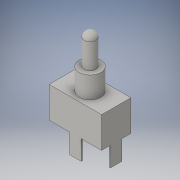
# Autodesk Inventor part: switch toggle
Saved by Autodesk Inventor 2016 (Build 200138000, 138)
## iProperties
Created: 2015-10-15
Part Number: switch toggle
Material: Generic
Document SubType Name: Modeling
Designer: jeremyhale
Density: 1 g/cm^3
Appearance: Default
Author: jeremyhale
Autodesk Inventor part; units mm, degrees
ref_plane "YZ Plane" through (0, 0, 0) normal (1, 0, 0) x (0, 1, 0)
ref_plane "XZ Plane" through (0, 0, 0) normal (0, 1, 0) x (-1, 0, 0)
ref_plane "XY Plane" through (0, 0, 0) normal (0, 0, 1) x (1, 0, 0)
sketch "Sketch1" plane through (0, 0, 0) normal (0, 1, 0) x (-1, 0, 0)
  line L0 (-14.4018, 8.0518) -> (14.4018, 8.0518)
  line L1 (14.4018, 8.0518) -> (14.4018, -8.0518)
  line L2 (14.4018, -8.0518) -> (-14.4018, -8.0518)
  line L3 (-14.4018, -8.0518) -> (-14.4018, 8.0518)
  line L4 (-14.4018, 8.0518) -> (14.4018, -8.0518) construction
  line L5 (14.4018, 8.0518) -> (-14.4018, -8.0518) construction
  point P0 (0, 0)
  dimension "d0" = 28.8036
  dimension "d1" = 16.1036
  constraints: 12 end point, 2 midpoint, 2 parallel, 1 horizontal, 1 perpendicular
  measures "d0" distance of L1.end L2.end
  measures "d1" distance of L0.end L1.end
extrude "Extrusion1" add sketch "Sketch1" along normal blind 17.018
sketch "Sketch2" plane through (0, 17.018, 0) normal (0, 1, 0) x (1, 0, 0)
  circle A0 centre (0, 0) radius 5.9531
  dimension "d4" = 11.9062
  constraints: 1 centre point, 1 coincident
  measures "d4" diameter of A0
extrude "Extrusion2" add sketch "Sketch2" along normal blind 11.811
sketch "Sketch3" plane through (0, 28.829, 0) normal (0, 1, 0) x (1, 0, 0)
  circle A0 centre (0, 0) radius 3.175
  dimension "d7" = 6.35
  constraints: 1 centre point, 1 coincident
  measures "d7" diameter of A0
extrude "Extrusion3" add sketch "Sketch3" along normal blind 16.9926
fillet "Fillet1" radius 3.175 1 edges at (-3.175, 45.8216, 0)
sketch "Sketch4" plane through (0, 0, 0) normal (0, -1, 0) x (1, 0, 0)
  line L0 (-14.4018, 8.0518) -> (14.4018, 8.0518) projected
  line L1 (0, 8.0518) -> (3.175, 8.0518)
  line L2 (3.175, 8.0518) -> (3.175, 7.2644)
  line L3 (3.175, 7.2644) -> (0, 7.2644)
  line L4 (0, 7.2644) -> (0, 8.0518)
  line L5 (0, 8.0518) -> (-3.175, 8.0518)
  line L6 (-3.175, 8.0518) -> (-3.175, 7.2644)
  line L7 (-3.175, 7.2644) -> (0, 7.2644)
  point P0 (0, 0)
  dimension "d11" = 3.175
  dimension "d12" = 0.7874
  constraints: 14 end point, 2 parallel, 2 symmetric about line, 1 horizontal, 1 midpoint, 1 perpendicular
  measures "d11" distance of L2.end L3.end
  measures "d12" distance of L1.end L2.end
extrude "Extrusion4" add sketch "Sketch4" along normal blind 10.795
sketch "Sketch5" plane through (0, 0, 0) normal (0, -1, 0) x (1, 0, 0)
  line L0 (14.4018, -8.0518) -> (14.4018, 8.0518) projected
  line L1 (14.4018, 0) -> (13.6144, 0)
  line L2 (13.6144, 0) -> (13.6144, 3.175)
  line L3 (13.6144, 3.175) -> (14.4018, 3.175)
  line L4 (14.4018, 3.175) -> (14.4018, 0)
  line L5 (13.6144, 0) -> (13.6144, -3.175)
  line L6 (13.6144, -3.175) -> (14.4018, -3.175)
  line L7 (14.4018, -3.175) -> (14.4018, 0)
  point P0 (0, 0)
  dimension "d15" = 0.7874
  dimension "d16" = 3.175
  constraints: 14 end point, 2 parallel, 2 symmetric about line, 1 horizontal, 1 midpoint, 1 perpendicular
  measures "d15" distance of L2.end L3.end
  measures "d16" distance of L1.end L2.end
extrude "Extrusion5" add sketch "Sketch5" along normal blind 10.795
body "Solid1"
